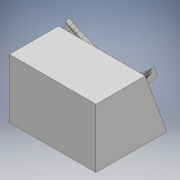
# Autodesk Inventor part: Supporto
Saved by Autodesk Inventor 2018 (Build 220112000, 112)
## iProperties
Created: 2020-01-18
Part Number: Supporto
Material: Generic
Document SubType Name: Modeling
Designer: Lorenzo Spadaro
Density: 1 g/cm^3
Appearance: Default
Author: Lorenzo Spadaro
Autodesk Inventor part; units mm, degrees
ref_plane "YZ Plane" through (0, 0, 0) normal (1, 0, 0) x (0, 1, 0)
ref_plane "XZ Plane" through (0, 0, 0) normal (0, 1, 0) x (-1, 0, 0)
ref_plane "XY Plane" through (0, 0, 0) normal (0, 0, 1) x (1, 0, 0)
sketch "Sketch1" plane through (0, 0, 0) normal (1, 0, 0) x (0, 1, 0)
  line L0 (0, 0) -> (0, 30)
  line L1 (0, 30) -> (25, 30)
  line L2 (25, 30) -> (35.9191, 0)
  line L3 (35.9191, 0) -> (0, 0)
  dimension "d0" = 30
  dimension "d1" = 25
  dimension "d3" = 70
  constraints: 8 end point, 1 horizontal, 1 perpendicular, 1 vertical
  measures "d0" distance of L0.start L0.end
  measures "d1" distance of L0.end L1.end
  measures "d3" angle of L2 L3
extrude "Extrusion1" add sketch "Sketch1" along normal blind 44
sketch "Sketch3" plane through (0, 25, 30) normal (0, 0.9396926, 0.3420201) x (1, 0, 0)
  line L0 (0.4638, 2.2659) -> (1.0416, 2.897)
  line L1 (1.0416, 2.897) -> (2.1956, 4.1576)
  line L2 (2.1956, 4.1576) -> (3.3774, 5.393)
  line L3 (3.3774, 5.393) -> (4.5847, 6.6043)
  line L4 (4.5847, 6.6043) -> (6.4389, 8.379)
  line L5 (6.4389, 8.379) -> (8.3381, 10.107)
  line L6 (8.3381, 10.107) -> (11.5828, 12.8945)
  line L7 (11.5828, 12.8945) -> (13.5652, 14.5186)
  line L8 (13.5652, 14.5186) -> (21.9997, 20.8165)
  line L9 (21.9997, 20.8165) -> (26.4814, 17.5559)
  line L10 (26.4814, 17.5559) -> (29.1299, 15.5365)
  line L11 (29.1299, 15.5365) -> (30.8721, 14.1594)
  line L12 (30.8721, 14.1594) -> (32.592, 12.7554)
  line L13 (32.592, 12.7554) -> (34.2866, 11.3219)
  line L14 (34.2866, 11.3219) -> (35.9526, 9.8571)
  line L15 (35.9526, 9.8571) -> (36.774, 9.1122)
  line L16 (36.774, 9.1122) -> (37.587, 8.3587)
  line L17 (37.587, 8.3587) -> (38.3914, 7.5962)
  line L18 (38.3914, 7.5962) -> (39.1867, 6.8245)
  line L19 (39.1867, 6.8245) -> (39.9726, 6.0433)
  line L20 (39.9726, 6.0433) -> (40.7488, 5.2523)
  line L21 (40.7488, 5.2523) -> (41.5146, 4.4513)
  line L22 (41.5146, 4.4513) -> (42.2698, 3.6401)
  line L23 (42.2698, 3.6401) -> (43.014, 2.8184)
  line L24 (43.014, 2.8184) -> (43.7468, 1.9857)
  line L25 (0, 31.9253) -> (44, 31.9253) projected
  line L26 (0, 0) -> (0, 31.9253) projected
  line L27 (44, 31.9253) -> (44, 0) projected
  line L28 (0, 0) -> (44, 0) projected
  line L29 (44, 31.9253) -> (22, 31.9253)
  line L30 (22, 28.8187) -> (22, -3.1066)
  line L31 (0.4638, 5.4706) -> (1.0417, 6.1017)
  line L32 (1.0417, 6.1017) -> (2.196, 7.362)
  line L33 (2.196, 7.362) -> (3.378, 8.5971)
  line L34 (3.378, 8.5971) -> (4.5856, 9.8082)
  line L35 (4.5856, 9.8082) -> (6.4401, 11.5826)
  line L36 (6.4401, 11.5826) -> (8.3396, 13.3102)
  line L37 (8.3396, 13.3102) -> (11.5849, 16.0971)
  line L38 (11.5849, 16.0971) -> (13.5676, 17.7208)
  line L39 (13.5676, 17.7208) -> (22.0034, 24.017)
  line L40 (22.0034, 24.017) -> (26.4845, 20.7555)
  line L41 (26.4845, 20.7555) -> (29.1325, 18.7356)
  line L42 (29.1325, 18.7356) -> (30.8745, 17.3582)
  line L43 (30.8745, 17.3582) -> (32.5941, 15.9538)
  line L44 (32.5941, 15.9538) -> (34.2883, 14.52)
  line L45 (34.2883, 14.52) -> (35.9541, 13.0549)
  line L46 (35.9541, 13.0549) -> (36.7753, 12.3098)
  line L47 (36.7753, 12.3098) -> (37.5882, 11.5561)
  line L48 (37.5882, 11.5561) -> (38.3925, 10.7934)
  line L49 (38.3925, 10.7934) -> (39.1876, 10.0216)
  line L50 (39.1876, 10.0216) -> (39.9734, 9.2402)
  line L51 (39.9734, 9.2402) -> (40.7494, 8.4491)
  line L52 (40.7494, 8.4491) -> (41.515, 7.6479)
  line L53 (41.515, 7.6479) -> (42.2701, 6.8366)
  line L54 (42.2701, 6.8366) -> (43.0141, 6.0147)
  line L55 (43.0141, 6.0147) -> (43.7468, 5.1818)
  line L56 (43.7468, 1.9857) -> (43.7468, 5.1818)
  line L57 (0.4638, 2.2659) -> (0.4638, 5.4706)
  point P0 (0, 19.6403)
  dimension "d4" = 44
  dimension "d5" = 0
  dimension "d6" = 22
  constraints: 108 end point, 2 parallel
  measures "d6" distance of L29.end L25.end
extrude "Extrusion2" add sketch "Sketch3" along normal blind 5 contours L57 L31 L32 L33 L34 L35 L36 L37 L38 L39 L30 L8 L7 L6 L5 L4 L3 L2 L1 L0 | L30 L39 L40 L41 L42 L43 L44 L45 L46 L47 L48 L49 L50 L51 L52 L53 L54 L55 L56 L24 L23 L22 L21 L20 L19 L18 L17 L16 L15 L14 L13 L12 L11 L10 L9
sketch "Sketch4" plane through (0, 29.6985, 31.7101) normal (0, 0.9396926, 0.3420201) x (1, 0, 0)
  line L0 (43.014, 2.8184) -> (43.7468, 1.9857) projected
  line L1 (42.2698, 3.6401) -> (43.014, 2.8184) projected
  line L2 (41.5146, 4.4513) -> (42.2698, 3.6401) projected
  line L3 (40.7488, 5.2523) -> (41.5146, 4.4513) projected
  line L4 (39.9726, 6.0433) -> (40.7488, 5.2523) projected
  line L5 (39.1867, 6.8245) -> (39.9726, 6.0433) projected
  line L6 (38.3914, 7.5962) -> (39.1867, 6.8245) projected
  line L7 (37.587, 8.3587) -> (38.3914, 7.5962) projected
  line L8 (36.774, 9.1122) -> (37.587, 8.3587) projected
  line L9 (35.9526, 9.8571) -> (36.774, 9.1122) projected
  line L10 (34.2866, 11.3219) -> (35.9526, 9.8571) projected
  line L11 (32.592, 12.7554) -> (34.2866, 11.3219) projected
  line L12 (30.8721, 14.1594) -> (32.592, 12.7554) projected
  line L13 (29.1299, 15.5365) -> (30.8721, 14.1594) projected
  line L14 (26.4814, 17.5559) -> (29.1299, 15.5365) projected
  line L15 (21.9997, 20.8165) -> (26.4814, 17.5559) projected
  line L16 (13.5652, 14.5186) -> (21.9997, 20.8165) projected
  line L17 (11.5828, 12.8945) -> (13.5652, 14.5186) projected
  line L18 (8.3381, 10.107) -> (11.5828, 12.8945) projected
  line L19 (6.4389, 8.379) -> (8.3381, 10.107) projected
  line L20 (4.5847, 6.6043) -> (6.4389, 8.379) projected
  line L21 (3.3774, 5.393) -> (4.5847, 6.6043) projected
  line L22 (2.1956, 4.1576) -> (3.3774, 5.393) projected
  line L23 (0.4638, 2.2659) -> (2.1956, 4.1576) projected
  line L24 (43.0095, 1.2134) -> (43.7468, 0.0915)
  line L25 (42.26, 2.0304) -> (43.0095, 1.2134)
  line L26 (41.4996, 2.8367) -> (42.26, 2.0304)
  line L27 (40.7286, 3.6327) -> (41.4996, 2.8367)
  line L28 (39.9474, 4.4186) -> (40.7286, 3.6327)
  line L29 (39.1564, 5.1947) -> (39.9474, 4.4186)
  line L30 (38.3561, 5.9612) -> (39.1564, 5.1947)
  line L31 (37.5468, 6.7185) -> (38.3561, 5.9612)
  line L32 (36.7289, 7.4668) -> (37.5468, 6.7185)
  line L33 (35.9027, 8.2064) -> (36.7289, 7.4668)
  line L34 (34.2272, 9.6603) -> (35.9027, 8.2064)
  line L35 (32.5234, 11.0828) -> (34.2272, 9.6603)
  line L36 (30.7945, 12.4757) -> (32.5234, 11.0828)
  line L37 (29.0434, 13.8414) -> (30.7945, 12.4757)
  line L38 (26.3819, 15.8436) -> (29.0434, 13.8414)
  line L39 (21.8791, 19.0751) -> (26.3819, 15.8436)
  line L40 (13.4856, 12.7228) -> (21.8791, 19.0751)
  line L41 (11.5138, 11.0859) -> (13.4856, 12.7228)
  line L42 (8.2871, 8.2775) -> (11.5138, 11.0859)
  line L43 (6.3992, 6.5372) -> (8.2871, 8.2775)
  line L44 (4.5566, 4.7505) -> (6.3992, 6.5372)
  line L45 (3.3571, 3.5314) -> (4.5566, 4.7505)
  line L46 (2.1833, 2.2884) -> (3.3571, 3.5314)
  line L47 (0.4638, 0.3855) -> (2.1833, 2.2884)
  line L48 (43.7468, 1.9857) -> (43.7468, 5.1818) projected
  line L49 (43.7468, 1.9857) -> (43.7468, 0.0915)
  line L50 (44, 31.9253) -> (44, 0) projected
  line L51 (0.4638, 2.2659) -> (0.4638, 0.3855)
  point P0 (0, 19.6403)
  point P1 (1, 20.6403)
  constraints: 52 end point, 2 parallel
extrude "Extrusion3" add sketch "Sketch4" against normal blind 2
body "Solid1"
